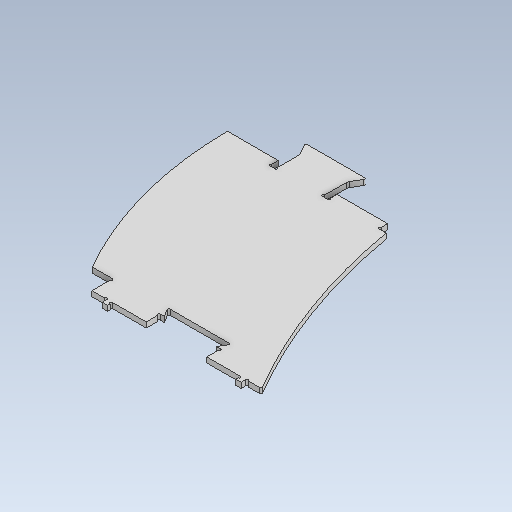
# Autodesk Inventor part: Support B
Saved by Autodesk Inventor 2020 (Build 240168000, 168)
## iProperties
Created: 2020-03-07
Part Number: Support B
Material: Generic
Document SubType Name: Modeling
Designer: Daniel Wikman
Density: 1 g/cm^3
Appearance: Default
Author: Daniel Wikman
Autodesk Inventor part; units mm, degrees
ref_plane "YZ Plane" through (0, 0, 0) normal (1, 0, 0) x (0, 1, 0)
ref_plane "XZ Plane" through (0, 0, 0) normal (0, 1, 0) x (-1, 0, 0)
ref_plane "XY Plane" through (0, 0, 0) normal (0, 0, 1) x (1, 0, 0)
sketch "Sketch1" plane through (0, 0, 0) normal (0, 1, 0) x (-1, 0, 0)
  line L0 (54.5284, -163.8048) -> (49.6951, -172.1764)
  arc A0 (49.6951, -172.1764) -> (50.8498, -174.1764) centre (50.8498, -172.843) ccw
  line L1 (50.8498, -174.1764) -> (117.5164, -174.1764)
  line L2 (113.8378, -163.8048) -> (118.6711, -172.1764)
  arc A1 (117.5164, -174.1764) -> (118.6711, -172.1764) centre (117.5164, -172.843) ccw
  arc A2 (259.3338, -380.9628) -> (202.7682, -171.3935) centre (-165.66, -383.2559) ccw
  line L3 (113.8378, -163.8048) -> (118.3961, -163.8048)
  arc A3 (118.3961, -163.8048) -> (118.4865, -161.1412) centre (118.3961, -162.4715) ccw
  line L4 (54.5284, -163.8048) -> (49.9178, -163.8048)
  arc A4 (49.9178, -161.1381) -> (49.9178, -163.8048) centre (49.9178, -162.4715) ccw
  line L5 (5.6828, -148.1362) -> (5.6828, -142.6365)
  line L6 (5.6828, -142.6365) -> (11.6828, -142.6364)
  line L7 (11.6828, -142.6364) -> (11.6828, -145.4697)
  arc A5 (11.6828, -145.4697) -> (11.6828, -148.1364) centre (11.6828, -146.803) ccw
  arc A6 (3.0183, -148.0602) -> (5.6828, -148.1362) centre (4.3494, -148.1362) ccw
  line L8 (162.7021, -148.1362) -> (162.7021, -142.6363)
  line L9 (162.7021, -142.6363) -> (156.7021, -142.6363)
  line L10 (156.7021, -142.6363) -> (156.7021, -145.4697)
  arc A7 (156.7021, -148.1364) -> (156.7021, -145.4697) centre (156.7021, -146.803) ccw
  arc A8 (162.7021, -148.1362) -> (165.3666, -148.0602) centre (164.0355, -148.1362) ccw
  line L11 (165.3666, -148.0602) -> (179.8476, -148.0602)
  line L12 (179.8476, -148.0602) -> (179.8476, -168.7268)
  arc A9 (179.8476, -168.7268) -> (179.8476, -171.3935) centre (179.8476, -170.0602) ccw
  line L13 (179.8476, -171.3935) -> (202.7682, -171.3935)
  line L14 (78.171, -370.9703) -> (69.785, -370.9703)
  line L15 (168.6888, -389.73) -> (168.6888, -432.7538)
  arc A10 (201.1888, -413.0028) -> (202.3435, -411.0028) centre (201.1888, -411.6694) ccw
  line L16 (195.5003, -397.8103) -> (195.5003, -373.6294)
  arc A11 (195.5003, -370.9628) -> (195.5003, -373.6294) centre (195.5003, -372.2961) ccw
  line L17 (195.5003, -370.9628) -> (202.0003, -370.9628)
  arc A12 (202.0003, -373.6294) -> (202.0003, -370.9628) centre (202.0003, -372.2961) ccw
  line L18 (202.0003, -373.6294) -> (202.0003, -380.9628)
  line L19 (78.1632, -380.9628) -> (135.4967, -380.9628)
  line L20 (202.0003, -380.9628) -> (259.3338, -380.9628)
  arc A13 (135.0341, -411.0028) -> (136.1888, -413.0028) centre (136.1888, -411.6694) ccw
  arc A14 (141.8773, -373.6233) -> (142.0056, -370.9628) centre (142.0056, -372.2961) ccw
  line L21 (142.0056, -370.9628) -> (135.5056, -370.9628)
  arc A15 (135.5056, -370.9628) -> (135.5032, -373.6294) centre (135.5056, -372.2961) ccw
  line L22 (135.5032, -373.6294) -> (135.4967, -380.9628)
  line L23 (49.9178, -161.1381) -> (49.9178, -148.1364)
  line L24 (118.4865, -148.1364) -> (118.4865, -161.1412)
  line L25 (202.3435, -411.0028) -> (196.1702, -400.3103)
  arc A16 (195.5003, -397.8103) -> (196.1702, -400.3103) centre (200.5003, -397.8103) ccw
  line L26 (141.8773, -397.8103) -> (141.8773, -373.6233)
  line L27 (135.0341, -411.0028) -> (141.2075, -400.3103)
  arc A17 (141.2075, -400.3103) -> (141.8773, -397.8103) centre (136.8773, -397.8103) ccw
  arc A18 (78.1697, -373.637) -> (78.171, -370.9703) centre (78.171, -372.3036) ccw
  line L28 (78.1632, -380.9628) -> (78.1697, -373.637)
  line L29 (136.1888, -413.0028) -> (201.1888, -413.0028)
  arc A19 (-9.9624, -148.0602) -> (-11.0329, -150.3848) centre (-9.9624, -149.469) ccw
  arc A20 (69.785, -370.9703) -> (-10.5152, -151.1127) centre (-579.254, -483.4304) ccw
  arc A21 (-10.5152, -151.1127) -> (-11.0329, -150.3848) centre (-14.8322, -153.6352) ccw
  line L30 (118.4865, -148.1364) -> (156.7021, -148.1364)
  line L31 (84.1831, -174.1764) -> (84.1831, -204.8832)
  line L32 (-9.9624, -148.0602) -> (3.0183, -148.0602)
  line L33 (11.6828, -148.1364) -> (49.9178, -148.1364)
  point P0 (2.7021, -144.053)
  point P1 (1.3688, -146.803)
  point P2 (-3.2979, -145.3864)
  point P3 (-7.9624, -148.0602)
  point P4 (116.117, -163.8048)
  dimension "d102" = 2.6667
  dimension "d107" = 2.6667
  dimension "d108" = 6.5
  dimension "d109" = 2.6667
  dimension "d111" = 57.3335
  dimension "d127" = 9.6667
  dimension "d128" = 9.6667
  dimension "d129" = 1.3333
  dimension "d131" = 62.3312
  dimension "d132" = 1.3333
  dimension "d133" = 14.481
  dimension "d134" = 1.3333
  dimension "d135" = 6
  dimension "d141" = 7.3333
  dimension "d142" = 5
  dimension "d145" = 1.3333
  dimension "d149" = 1.3333
  dimension "d151" = 658.71
  dimension "d152" = 5
  dimension "d153" = 68.5687
  dimension "d154" = 66.6667
  dimension "d155" = 1.3333
  dimension "d156" = 1.3333
  dimension "d158" = 1.3333
  dimension "d160" = 10.3716
  dimension "d161" = 10.3716
  dimension "d162" = 38.2156
  dimension "d163" = 38.235
  dimension "d164" = 15.6684
  dimension "d165" = 15.6684
  dimension "d166" = 23.3333
  dimension "d167" = 84.5058
  dimension "d169" = 264.8664
  dimension "d170" = 145.0381
  dimension "d171" = 6
  dimension "d172" = 5.4997
  dimension "d173" = 1.3333
  dimension "d174" = 2.8333
  dimension "d175" = 145.0006
  constraints: 68 end point, 45 point on circle, 22 centre point, 12 tangent, 8 horizontal, 4 point on line, 3 symmetric about line, 2 midpoint, 2 vertical, 1 collinear, 5 other
  measures "d102" diameter of A10
  measures "d107" diameter of A11
  measures "d108" distance of L17.start L17.end
  measures "d109" diameter of A12
  measures "d111" distance of L19.start L19.end
  measures "d127" distance of L2.start L2.end
  measures "d128" distance of L0.start L0.end
  measures "d129" radius of A1
  measures "d131" distance from line of A1.centre L12
  measures "d132" radius of A9
  measures "d133" distance of L11.start L11.end
  measures "d134" radius of A8
  measures "d135" distance between parallel lines of L10 L8
  measures "d141" distance of L18.start L18.end
  measures "d142" radius of A16
  measures "d145" radius of A5
  measures "d149" radius of A18
  measures "d151" radius of A20
  measures "d152" radius of A21
  measures "d153" distance between parallel lines of L23 L24
  measures "d154" distance of L1.start L1.end
  measures "d155" radius of A0
  measures "d156" radius of A4
  measures "d158" radius of A3
  measures "d160" distance between parallel lines of L1 L4
  measures "d161" distance between parallel lines of L1 L3
  measures "d162" distance from line of L30.end L24
  measures "d163" distance from line of L33.start L23
  measures "d164" distance from line of L23.end L4
  measures "d165" distance from line of L24.start L3
  measures "d166" distance between parallel lines of L13 L11
  measures "d167" distance between parallel lines of L15 L31
  measures "d169" distance between parallel lines of L30 L29
  measures "d170" diameter of L10.start L31
  measures "d171" distance of L5.end L6.end
  measures "d172" distance of L5.start L5.end
  measures "d173" radius of A6
  measures "d174" distance of L6.end L7.end
  measures "d175" diameter of L6.end L31
extrude "Extrusion3" add sketch "Sketch1" along normal blind 6
body "Solid3"
